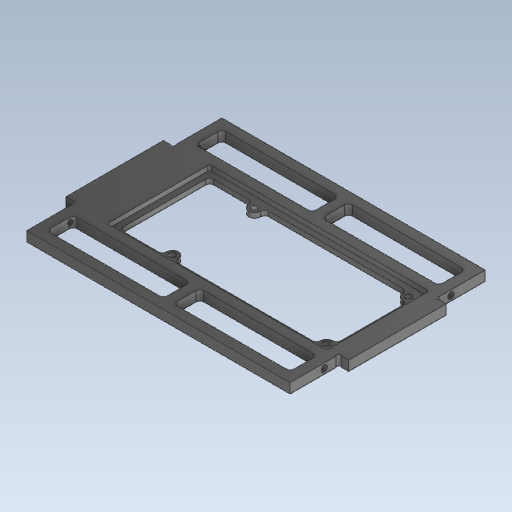
# Autodesk Inventor part: Cockpit_carrier_board_frame
Saved by Autodesk Inventor 2020.4 (Build 244396000, 396)
## iProperties
Created: 2022-01-28
Part Number: Cockpit_carrier_board_frame
Material: アセタール樹脂、黒
Document SubType Name: Modeling
Designer: Masato Kubotera
Density: 1.425 g/cm^3
Appearance: 滑らか - 黒
Author: Masato Kubotera
Autodesk Inventor part; units mm, degrees
ref_plane "YZ Plane" through (0, 0, 0) normal (1, 0, 0) x (0, 1, 0)
derived "Cockpit_side_frame.ipt"
sketch "スケッチ2" plane through (0, 0, 0) normal (0, 1, 0) x (-1, 0, 0)
  line L0 (-28.5, -22.5) -> (86.5, -22.5) construction
  line L1 (86.5, -22.5) -> (86.5, -138.5)
  line L2 (86.5, -96) -> (-28.5, -96) construction
  line L3 (-28.5, -96) -> (-28.5, -22.5) construction
  line L4 (-28.5, -22.5) -> (86.5, -96) construction
  line L5 (86.5, -22.5) -> (-28.5, -96) construction
  line L6 (36.5, -101) -> (36.5, -133.5)
  line L7 (41.5, -138.5) -> (86.5, -138.5)
  arc A0 (62.6349, -70.4) -> (61.15, -71.8849) centre (61.8925, -71.1425) ccw
  arc A1 (71.15, -72.5349) -> (69.6651, -71.05) centre (70.4075, -71.7925) ccw
  line L8 (63.3349, -71.05) -> (69.6651, -71.05)
  line L9 (62.6349, -70.4) -> (70.3651, -70.4)
  line L10 (61.9, -71.1) -> (71.1, -71.1) construction
  arc A2 (63.3349, -71.05) -> (61.85, -72.5349) centre (62.5925, -71.7925) ccw
  line L11 (61.2, -70.45) -> (71.8, -70.45) construction
  line L12 (71.15, -72.5349) -> (71.15, -83.4651)
  line L13 (71.8, -78) -> (61.2, -78) construction
  line L14 (71.85, -71.8849) -> (71.85, -84.1151)
  line L15 (71.1, -71.1) -> (71.1, -84.9) construction
  line L16 (61.85, -72.5349) -> (61.85, -83.4651)
  line L17 (71.8, -70.45) -> (71.8, -85.55) construction
  line L18 (61.15, -71.8849) -> (61.15, -84.1151)
  line L19 (66.5, -70.45) -> (66.5, -85.55) construction
  line L20 (61.9, -84.9) -> (61.9, -71.1) construction
  line L21 (71.1, -71.1) -> (61.9, -84.9) construction
  line L22 (71.8, -70.45) -> (61.2, -85.55) construction
  line L23 (61.2, -70.45) -> (71.8, -85.55) construction
  line L24 (61.2, -85.55) -> (61.2, -70.45) construction
  line L25 (61.9, -71.1) -> (71.1, -84.9) construction
  arc A3 (71.85, -71.8849) -> (70.3651, -70.4) centre (71.1075, -71.1425) ccw
  line L26 (71.1, -84.9) -> (61.9, -84.9) construction
  line L27 (71.8, -85.55) -> (61.2, -85.55) construction
  arc A4 (61.85, -83.4651) -> (63.3349, -84.95) centre (62.5925, -84.2075) ccw
  arc A5 (61.15, -84.1151) -> (62.6349, -85.6) centre (61.8925, -84.8575) ccw
  line L28 (63.3349, -84.95) -> (69.6651, -84.95)
  line L29 (62.6349, -85.6) -> (70.3651, -85.6)
  arc A6 (69.6651, -84.95) -> (71.15, -83.4651) centre (70.4075, -84.2075) ccw
  arc A7 (70.3651, -85.6) -> (71.85, -84.1151) centre (71.1075, -84.8575) ccw
  line L30 (-23.5, -22.5) -> (-28.5, -27.5)
  line L31 (-28.5, -59.25) -> (86.5, -59.25) construction
  line L32 (29, -22.5) -> (29, -96) construction
  line L33 (-23.5, -96) -> (-28.5, -91)
  line L34 (-28.5, -27.5) -> (-28.5, -91)
  line L35 (-21, -25) -> (-26, -25) construction
  line L36 (-26, -25) -> (-26, -93.5) construction
  line L37 (-26, -93.5) -> (-21, -93.5) construction
  line L38 (-21, -93.5) -> (-21, -25) construction
  line L39 (-21, -25) -> (-26, -93.5) construction
  line L40 (-26, -25) -> (-21, -93.5) construction
  line L41 (-26.05, -46.7) -> (-20.95, -46.7)
  line L42 (-20.95, -46.7) -> (-20.95, -71.8)
  line L43 (-20.95, -71.8) -> (-26.05, -71.8)
  line L44 (-26.05, -71.8) -> (-26.05, -46.7)
  line L45 (-26.05, -46.7) -> (-20.95, -71.8) construction
  line L46 (-20.95, -46.7) -> (-26.05, -71.8) construction
  line L47 (-26, -46.75) -> (-21, -46.75) construction
  line L48 (-26, -71.75) -> (-21, -71.75) construction
  line L49 (-23.5, -25) -> (-23.5, -93.5) construction
  circle A8 centre (-23.5, -35) radius 3
  circle A9 centre (-23.5, -35) radius 1.6
  arc A10 (-24.5651, -46.7) -> (-26.05, -48.1849) centre (-25.3075, -47.4425) ccw
  arc A11 (-20.95, -48.1849) -> (-22.4349, -46.7) centre (-21.6925, -47.4425) ccw
  arc A12 (-22.4349, -71.8) -> (-20.95, -70.3151) centre (-21.6925, -71.0575) ccw
  arc A13 (-26.05, -70.3151) -> (-24.5651, -71.8) centre (-25.3075, -71.0575) ccw
  circle A14 centre (-23.5, -83.5) radius 1.6
  circle A15 centre (-23.5, -83.5) radius 3
  line L50 (31.5, -96) -> (36.5, -101)
  line L51 (-23.5, -96) -> (31.5, -96)
  line L52 (79, -67.5) -> (-21, -67.5) construction
  line L53 (-21, -67.5) -> (-21, -62.5) construction
  line L54 (-21, -62.5) -> (79, -62.5) construction
  line L55 (79, -62.5) -> (79, -67.5) construction
  line L56 (79, -67.5) -> (-21, -62.5) construction
  line L57 (-21, -67.5) -> (79, -62.5) construction
  line L58 (-21, -65) -> (79, -65) construction
  line L59 (29, -62.5) -> (29, -67.5) construction
  line L60 (4, -62.5) -> (4, -67.5) construction
  line L61 (54.05, -62.45) -> (3.95, -62.45)
  line L62 (3.95, -62.45) -> (3.95, -67.55)
  line L63 (3.95, -67.55) -> (54.05, -67.55)
  line L64 (54.05, -67.55) -> (54.05, -62.45)
  line L65 (54.05, -62.45) -> (3.95, -67.55) construction
  line L66 (3.95, -62.45) -> (54.05, -67.55) construction
  arc A16 (5.4349, -62.45) -> (3.95, -63.9349) centre (4.6925, -63.1925) ccw
  circle A17 centre (-3.5, -65) radius 3
  circle A18 centre (-3.5, -65) radius 1.6
  line L67 (54, -62.5) -> (54, -67.5) construction
  arc A19 (54.05, -63.9349) -> (52.5651, -62.45) centre (53.3075, -63.1925) ccw
  circle A20 centre (61.5, -65) radius 3
  circle A21 centre (61.5, -65) radius 1.6
  arc A22 (3.95, -66.0651) -> (5.4349, -67.55) centre (4.6925, -66.8075) ccw
  arc A23 (52.5651, -67.55) -> (54.05, -66.0651) centre (53.3075, -66.8075) ccw
  line L68 (-21, -88.5) -> (79, -88.5) construction
  line L69 (79, -88.5) -> (79, -93.5) construction
  line L70 (79, -93.5) -> (-21, -93.5) construction
  line L71 (-21, -93.5) -> (-21, -88.5) construction
  line L72 (-21, -88.5) -> (79, -93.5) construction
  line L73 (79, -88.5) -> (-21, -93.5) construction
  line L74 (-21, -91) -> (79, -91) construction
  line L75 (29, -88.5) -> (29, -93.5) construction
  line L76 (54.05, -91.05) -> (3.95, -91.05)
  line L77 (3.95, -91.05) -> (3.95, -88.45)
  line L78 (3.95, -88.45) -> (54.05, -88.45)
  line L79 (54.05, -88.45) -> (54.05, -91.05)
  line L80 (54.05, -91.05) -> (3.95, -88.45) construction
  line L81 (3.95, -91.05) -> (54.05, -88.45) construction
  line L82 (4, -88.5) -> (4, -91) construction
  line L83 (54, -88.5) -> (54, -91) construction
  line L84 (4, -89.75) -> (54, -89.75) construction
  arc A24 (6.05, -88.45) -> (3.95, -88.45) centre (5, -88.45) ccw
  arc A25 (54.05, -88.45) -> (51.95, -88.45) centre (53, -88.45) ccw
  arc A26 (51.95, -91.05) -> (54.05, -91.05) centre (53, -91.05) ccw
  arc A27 (3.95, -91.05) -> (6.05, -91.05) centre (5, -91.05) ccw
  circle A28 centre (-3.5, -91) radius 3
  circle A29 centre (-3.5, -91) radius 1.6
  circle A30 centre (61.5, -91) radius 3 construction
  circle A31 centre (61.5, -91) radius 1.6 construction
  line L85 (-23.5, -22.5) -> (64.25, -22.5)
  line L86 (64.25, -22.5) -> (64.25, -17.5)
  line L87 (64.25, -17.5) -> (72.25, -17.5)
  line L88 (72.25, -17.5) -> (72.25, -22.5)
  line L89 (72.25, -22.5) -> (79, -22.5)
  line L90 (79, -22.5) -> (79, -17.5)
  line L91 (86.5, -22.5) -> (86.5, -20)
  line L92 (79, -17.5) -> (84, -17.5)
  line L93 (84, -17.5) -> (86.5, -20)
  line L94 (68.25, -17.5) -> (68.25, -22.5) construction
  arc A32 (62.7651, -22.5) -> (64.25, -21.0151) centre (63.5075, -21.7575) ccw
  arc A33 (72.25, -21.0151) -> (73.7349, -22.5) centre (72.9925, -21.7575) ccw
  arc A34 (77.5151, -22.5) -> (79, -21.0151) centre (78.2575, -21.7575) ccw
  line L95 (-16, -88.5) -> (-16, -68.5) construction
  line L96 (-16, -68.5) -> (64, -68.5) construction
  line L97 (64, -68.5) -> (64, -88.5) construction
  line L98 (45.5, -86) -> (-16.5, -86)
  line L99 (-18.5, -84) -> (-18.5, -72)
  line L100 (-16.5, -70) -> (45.5, -70)
  line L101 (47.5, -72) -> (47.5, -84)
  line L102 (47.5, -86) -> (-18.5, -70) construction
  line L103 (-18.5, -86) -> (47.5, -70) construction
  arc A35 (-16.5, -70) -> (-18.5, -72) centre (-16.5, -72) ccw
  arc A36 (-18.5, -84) -> (-16.5, -86) centre (-16.5, -84) ccw
  arc A37 (45.5, -86) -> (47.5, -84) centre (45.5, -84) ccw
  arc A38 (47.5, -72) -> (45.5, -70) centre (45.5, -72) ccw
  line L104 (36.5, -133.5) -> (41.5, -138.5)
  line L105 (44, -131) -> (39, -131) construction
  line L106 (39, -131) -> (39, -96) construction
  line L107 (39, -96) -> (44, -96) construction
  line L108 (44, -96) -> (44, -131) construction
  line L109 (44, -131) -> (39, -96) construction
  line L110 (39, -131) -> (44, -96) construction
  line L111 (41.5, -96) -> (41.5, -131) construction
  line L112 (39, -113.5) -> (44, -113.5) construction
  line L113 (41.5, -107.5) -> (44, -107.5) construction
  line L114 (41.45, -107.45) -> (44.05, -107.45)
  line L115 (44.05, -107.45) -> (44.05, -119.55)
  line L116 (44.05, -119.55) -> (41.45, -119.55)
  line L117 (41.45, -119.55) -> (41.45, -107.45)
  line L118 (41.45, -107.45) -> (44.05, -119.55) construction
  line L119 (44.05, -107.45) -> (41.45, -119.55) construction
  arc A39 (44.05, -109.55) -> (44.05, -107.45) centre (44.05, -108.5) ccw
  arc A40 (42.9349, -107.45) -> (41.45, -108.9349) centre (42.1925, -108.1925) ccw
  arc A41 (44.05, -119.55) -> (44.05, -117.45) centre (44.05, -118.5) ccw
  line L120 (41.5, -119.5) -> (44, -119.5) construction
  arc A42 (41.45, -118.0651) -> (42.9349, -119.55) centre (42.1925, -118.8075) ccw
  line L121 (42.75, -107.5) -> (42.75, -119.5) construction
  circle A43 centre (41.5, -125.5) radius 3 construction
  circle A44 centre (41.5, -125.5) radius 1.6 construction
  circle A45 centre (41.5, -101.5) radius 3
  circle A46 centre (41.5, -101.5) radius 1.6
  circle A47 centre (-13.5, -55) radius 2
  line L122 (39, -131) -> (77.8645, -131) construction
  line L123 (77.8645, -131) -> (77.8645, -136) construction
  line L124 (77.8645, -136) -> (39, -136) construction
  line L125 (39, -136) -> (39, -131) construction
  line L126 (39, -131) -> (77.8645, -136) construction
  line L127 (77.8645, -131) -> (39, -136) construction
  line L128 (39, -133.5) -> (77.8645, -133.5) construction
  line L129 (58.4322, -131) -> (58.4322, -136) construction
  line L130 (58.4322, -133.5) -> (58.4322, -131) construction
  line L131 (50.8822, -130.95) -> (65.9822, -130.95)
  line L132 (65.9822, -130.95) -> (65.9822, -133.55)
  line L133 (65.9822, -133.55) -> (50.8822, -133.55)
  line L134 (50.8822, -133.55) -> (50.8822, -130.95)
  line L135 (50.8822, -130.95) -> (65.9822, -133.55) construction
  line L136 (65.9822, -130.95) -> (50.8822, -133.55) construction
  line L137 (50.9322, -131) -> (50.9322, -133.5) construction
  arc A48 (52.9822, -130.95) -> (50.8822, -130.95) centre (51.9322, -130.95) ccw
  arc A49 (50.8822, -132.0651) -> (52.3672, -133.55) centre (51.6247, -132.8075) ccw
  arc A50 (65.9822, -130.95) -> (63.8822, -130.95) centre (64.9322, -130.95) ccw
  arc A51 (64.4973, -133.55) -> (65.9822, -132.0651) centre (65.2398, -132.8075) ccw
  line L138 (65.9322, -131) -> (65.9322, -133.5) construction
  line L139 (50.9322, -132.25) -> (65.9322, -132.25) construction
  circle A52 centre (72.4322, -133.5) radius 1.6 construction
  circle A53 centre (72.4322, -133.5) radius 3 construction
  circle A54 centre (44.4322, -133.5) radius 3
  circle A55 centre (44.4322, -133.5) radius 1.6
  line L140 (48.5, -96) -> (77, -96)
  line L141 (79, -98) -> (79, -126.5)
  line L142 (77, -128.5) -> (48.5, -128.5)
  line L143 (46.5, -126.5) -> (46.5, -98)
  line L144 (46.5, -96) -> (79, -128.5) construction
  line L145 (79, -96) -> (46.5, -128.5) construction
  arc A56 (48.5, -96) -> (46.5, -98) centre (48.5, -98) ccw
  arc A57 (46.5, -126.5) -> (48.5, -128.5) centre (48.5, -126.5) ccw
  arc A58 (77, -128.5) -> (79, -126.5) centre (77, -126.5) ccw
  arc A59 (79, -98) -> (77, -96) centre (77, -98) ccw
  line L146 (79, -91.1738) -> (84, -91.1738) construction
  line L147 (84, -91.1738) -> (84, -136) construction
  line L148 (84, -136) -> (79, -136) construction
  line L149 (79, -136) -> (79, -91.1738) construction
  line L150 (79, -91.1738) -> (84, -136) construction
  line L151 (84, -91.1738) -> (79, -136) construction
  line L152 (81.5, -91.1738) -> (81.5, -136) construction
  circle A60 centre (81.5, -93.6738) radius 1.475
  circle A61 centre (81.5, -98.6738) radius 1.475
  circle A62 centre (81.5, -103.6738) radius 1.475
  circle A63 centre (81.5, -133.5) radius 1.6
  arc A64 (84, -91.1738) -> (79, -91.1738) centre (81.5, -133.5) ccw construction
  arc A65 (84.0111, -91.0742) -> (78.9889, -91.0742) centre (81.5, -133.5) ccw construction
  line L153 (86.5, -133.5) -> (81.5, -138.5)
  arc A66 (79, -131) -> (84, -136) centre (81.5, -133.5) ccw construction
  line L154 (79, -65) -> (84, -65) construction
  line L155 (84, -65) -> (84, -91) construction
  line L156 (84, -91) -> (79, -91) construction
  line L157 (79, -91) -> (79, -65) construction
  line L158 (79, -65) -> (84, -91) construction
  line L159 (84, -65) -> (79, -91) construction
  line L160 (79, -78) -> (84, -78) construction
  line L161 (81.5, -65) -> (81.5, -91) construction
  line L162 (79, -73) -> (84, -73) construction
  line L163 (78.95, -72.95) -> (86.5, -72.95)
  line L164 (84.05, -72.95) -> (84.05, -83.05) construction
  line L165 (84.05, -83.05) -> (78.95, -83.05)
  line L166 (78.95, -83.05) -> (78.95, -72.95)
  line L167 (78.95, -72.95) -> (84.05, -83.05) construction
  line L168 (84.05, -72.95) -> (78.95, -83.05) construction
  arc A67 (80.4349, -72.95) -> (78.95, -74.4349) centre (79.6925, -73.6925) ccw
  arc A68 (78.95, -81.5651) -> (80.4349, -83.05) centre (79.6925, -82.3075) ccw
  line L169 (79, -83) -> (84, -83) construction
  circle A69 centre (81.5, -68) radius 1.6
  circle A70 centre (81.5, -68) radius 3
  circle A71 centre (81.5, -88) radius 1.6
  circle A72 centre (81.5, -88) radius 3
  line L170 (84.05, -83.05) -> (86.5, -83.05)
  circle A73 centre (81.5, -133.5) radius 3
  line L171 (75.625, -22.5) -> (75.625, -27.147) construction
  line L172 (60.875, -22.5) -> (60.875, -27.147) construction
  line L173 (64.25, -22.5) -> (72.25, -22.5)
  point P0 (0, 0)
  point P1 (29, -59.25)
  point P2 (-25.7227, -96)
  point P3 (61.85, -71.05)
  point P4 (61.15, -70.4)
  point P5 (66.5, -78)
  point P6 (-23.5, -59.25)
  point P7 (29, -65)
  point P8 (29, -91)
  point P9 (29, -89.75)
  point P10 (29, -89.75)
  point P11 (52.5, -22)
  point P12 (14.5, -78)
  point P13 (-18.5, -61)
  point P14 (47.5, -61)
  point P15 (41.5, -113.5)
  point P16 (42.75, -113.5)
  point P17 (58.4322, -133.5)
  point P18 (58.4322, -132.25)
  point P19 (62.75, -112.25)
  point P20 (81.5, -113.5869)
  point P21 (81.5, -78)
  dimension "d1" = 67.5
  dimension "d2" = 5
  measures "d1" vertical distance of L52.start point (0, 0)
  measures "d2" distance of L54.end L52.start
ref_plane "作業平面1" through (0, 0, -67.5) normal (0, 0, 1) x (1, 0, 0)
sketch "スケッチ3" plane through (0, 0, -67.5) normal (0, 0, 1) x (1, 0, 0)
  line L0 (21, 0) -> (-79, 0) construction
  line L1 (-79, 0) -> (-79, -135)
  line L2 (-79, -135) -> (21, -135) construction
  line L3 (21, -135) -> (21, 0)
  line L4 (21, 0) -> (-79, -135) construction
  line L5 (-79, 0) -> (21, -135) construction
  line L6 (-4, 0) -> (-4, 5)
  line L7 (-4, 5) -> (-54, 5)
  line L8 (-54, 5) -> (-54, 0)
  arc A0 (-4, 1.4849) -> (-2.5151, 0) centre (-3.2575, 0.7425) ccw
  line L9 (-29, 0) -> (-29, -135) construction
  line L10 (21, -67.5) -> (-79, -67.5) construction
  arc A1 (-55.4849, 0) -> (-54, 1.4849) centre (-54.7425, 0.7425) ccw
  line L11 (-2.75, -117.5) -> (-55.25, -117.5)
  line L12 (-55.25, -117.5) -> (-55.25, -5)
  line L13 (-55.25, -5) -> (-2.75, -5)
  line L14 (-2.75, -5) -> (-2.75, -117.5)
  line L15 (-2.75, -117.5) -> (-55.25, -5) construction
  line L16 (-55.25, -117.5) -> (-2.75, -5) construction
  line L17 (-29, -5) -> (-29, -117.5) construction
  line L18 (-4, -6.25) -> (-54, -6.25) construction
  line L19 (-54, -6.25) -> (-54, -116.25) construction
  line L20 (-54, -116.25) -> (-4, -116.25) construction
  line L21 (-4, -116.25) -> (-4, -6.25) construction
  line L22 (-4, -6.25) -> (-54, -116.25) construction
  line L23 (-54, -6.25) -> (-4, -116.25) construction
  line L24 (-8, -89.25) -> (-50, -89.25) construction
  line L25 (-50, -89.25) -> (-50, -10.25) construction
  line L26 (-50, -10.25) -> (-8, -10.25) construction
  line L27 (-8, -10.25) -> (-8, -89.25) construction
  line L28 (-8, -89.25) -> (-50, -10.25) construction
  line L29 (-50, -89.25) -> (-8, -10.25) construction
  circle A2 centre (-50, -10.25) radius 1.6
  circle A3 centre (-50, -89.25) radius 1.6
  circle A4 centre (-8, -10.25) radius 1.6
  circle A5 centre (-8, -89.25) radius 1.6
  arc A6 (-50.15, -13.2462) -> (-47.0038, -10.1) centre (-50, -10.25) ccw
  line L30 (-45.0063, -8) -> (-12.9937, -8)
  arc A7 (-50.15, -92.2462) -> (-50.15, -86.2538) centre (-50, -89.25) ccw
  line L31 (-52.25, -94.2437) -> (-52.25, -112.5)
  line L32 (-50.25, -114.5) -> (-7.75, -114.5)
  line L33 (-52.25, -15.2437) -> (-52.25, -84.2563)
  arc A8 (-10.9962, -10.1) -> (-7.85, -13.2462) centre (-8, -10.25) ccw
  arc A9 (-7.85, -86.2538) -> (-7.85, -92.2462) centre (-8, -89.25) ccw
  line L34 (-5.75, -94.2437) -> (-5.75, -112.5)
  line L35 (-5.75, -15.2437) -> (-5.75, -84.2563)
  arc A10 (-45.0063, -8) -> (-47.0038, -10.1) centre (-45.0063, -10) ccw
  arc A11 (-50.15, -13.2462) -> (-52.25, -15.2437) centre (-50.25, -15.2437) ccw
  arc A12 (-52.25, -84.2563) -> (-50.15, -86.2538) centre (-50.25, -84.2563) ccw
  arc A13 (-50.15, -92.2462) -> (-52.25, -94.2437) centre (-50.25, -94.2437) ccw
  arc A14 (-52.25, -112.5) -> (-50.25, -114.5) centre (-50.25, -112.5) ccw
  arc A15 (-7.75, -114.5) -> (-5.75, -112.5) centre (-7.75, -112.5) ccw
  arc A16 (-5.75, -94.2437) -> (-7.85, -92.2462) centre (-7.75, -94.2437) ccw
  arc A17 (-7.85, -86.2538) -> (-5.75, -84.2563) centre (-7.75, -84.2563) ccw
  arc A18 (-10.9962, -10.1) -> (-12.9937, -8) centre (-12.9937, -10) ccw
  arc A19 (-5.75, -15.2437) -> (-7.85, -13.2462) centre (-7.75, -15.2437) ccw
  line L36 (-79, 0) -> (-55.4849, 0)
  line L37 (-2.5151, 0) -> (21, 0)
  line L38 (-4, -135) -> (-4, -140)
  line L39 (-4, -140) -> (-54, -140)
  line L40 (-54, -140) -> (-54, -135)
  arc A20 (-2.5151, -135) -> (-4, -136.4849) centre (-3.2575, -135.7425) ccw
  line L41 (-79, -135) -> (-55.4849, -135)
  line L42 (-2.5151, -135) -> (21, -135)
  line L43 (14, -65) -> (4.25, -65)
  line L44 (2.25, -63) -> (2.25, -7)
  line L45 (4.25, -5) -> (14, -5)
  line L46 (16, -7) -> (16, -63)
  line L47 (16, -65) -> (2.25, -5) construction
  line L48 (2.25, -65) -> (16, -5) construction
  arc A21 (4.25, -5) -> (2.25, -7) centre (4.25, -7) ccw
  arc A22 (2.25, -63) -> (4.25, -65) centre (4.25, -63) ccw
  arc A23 (14, -65) -> (16, -63) centre (14, -63) ccw
  arc A24 (16, -7) -> (14, -5) centre (14, -7) ccw
  line L49 (14, -70) -> (4.25, -70)
  line L50 (2.25, -72) -> (2.25, -128)
  line L51 (4.25, -130) -> (14, -130)
  line L52 (16, -128) -> (16, -72)
  arc A25 (2.25, -128) -> (4.25, -130) centre (4.25, -128) ccw
  arc A26 (4.25, -70) -> (2.25, -72) centre (4.25, -72) ccw
  arc A27 (16, -72) -> (14, -70) centre (14, -72) ccw
  arc A28 (14, -130) -> (16, -128) centre (14, -128) ccw
  line L53 (-72, -65) -> (-62.25, -65)
  line L54 (-60.25, -63) -> (-60.25, -7)
  line L55 (-62.25, -5) -> (-72, -5)
  line L56 (-74, -7) -> (-74, -63)
  arc A29 (-60.25, -7) -> (-62.25, -5) centre (-62.25, -7) ccw
  arc A30 (-62.25, -65) -> (-60.25, -63) centre (-62.25, -63) ccw
  arc A31 (-72, -5) -> (-74, -7) centre (-72, -7) ccw
  line L57 (-62.25, -130) -> (-72, -130)
  arc A32 (-62.25, -130) -> (-60.25, -128) centre (-62.25, -128) ccw
  arc A33 (-74, -128) -> (-72, -130) centre (-72, -128) ccw
  line L58 (-74, -128) -> (-74, -72)
  line L59 (-60.25, -72) -> (-60.25, -128)
  arc A34 (-72, -70) -> (-74, -72) centre (-72, -72) ccw
  line L60 (-72, -70) -> (-62.25, -70)
  arc A35 (-60.25, -72) -> (-62.25, -70) centre (-62.25, -72) ccw
  arc A36 (-54, -136.4849) -> (-55.4849, -135) centre (-54.7425, -135.7425) ccw
  arc A37 (-74, -63) -> (-72, -65) centre (-72, -63) ccw
  point P0 (0, 0)
  point P1 (-54, 1.4849)
  point P2 (-55.4849, 0)
  point P3 (-29, -61.25)
  point P4 (-29, -61.25)
  point P5 (-29, -49.75)
  point P6 (-52.25, -12.2343)
  point P7 (-48.0157, -8)
  point P8 (-52.25, -91.2343)
  point P9 (-52.25, -87.2657)
  point P10 (-52.25, -114.5)
  point P11 (-5.75, -12.2343)
  point P12 (-9.9843, -8)
  point P13 (-5.75, -91.2343)
  point P14 (-5.75, -87.2657)
  point P15 (-5.75, -114.5)
  point P16 (9.125, -35)
  dimension "d4" = 5
  dimension "d5" = 135
  dimension "d6" = 1.05
  dimension "d27" = 110
  dimension "d28" = 50
  dimension "d29" = 42
  dimension "d30" = 4
  dimension "d31" = 79
  dimension "d32" = 1.25
  dimension "d33" = 1.25
  dimension "d34" = 1.25
  dimension "d35" = 3.2
  dimension "d36" = 3.2
  dimension "d38" = 3
  dimension "d39" = 3
  dimension "d40" = 3
  dimension "d41" = 3
  dimension "d42" = 3
  dimension "d43" = 2
  dimension "d44" = 5
  dimension "d45" = 0
  dimension "d46" = 5
  dimension "d47" = 5
  dimension "d48" = 5
  dimension "d49" = 2.5
  dimension "d50" = 2
  constraints: 122 end point, 77 point on circle, 68 symmetric about line, 38 centre point, 28 tangent, 26 point on line, 15 midpoint, 12 equal radius, 12 parallel, 10 coincident, 8 perpendicular, 6 horizontal, 3 collinear, 1 vertical, 19 other
  measures "d4" distance of L6.start L6.end
  measures "d5" distance of L2.end L0.start
  measures "d6" radius of A0
  measures "d27" distance of L20.end L18.start
  measures "d28" distance of L18.start L18.end
  measures "d29" distance of L25.end L26.end
  measures "d30" horizontal distance of L18.end L25.end
  measures "d31" distance of L24.end L25.end
  measures "d32" horizontal distance of L12.end L18.end
  measures "d33" horizontal distance of L11.end L19.end
  measures "d34" horizontal distance of L12.end L18.end
  measures "d35" diameter of A2
  measures "d36" diameter of A3
  measures "d38" horizontal distance of L11.end point (-52.25, -114.5)
  measures "d39" horizontal distance of L11.end point (-52.25, -114.5)
  measures "d40" vertical distance of point (-48.016, -8) L12.end
  measures "d41" radius of A7
  measures "d42" radius of A6
  measures "d43" radius of A10
  measures "d44" vertical distance of L0.start L13.end
  measures "d45" horizontal distance of L9.start L17.start
  measures "d46" horizontal distance of L0.start L48.end
  measures "d47" distance of L13.end L47.end
  measures "d48" horizontal distance of L48.end L0.start
  measures "d49" vertical distance of L10.start L47.start
  measures "d50" radius of A21
extrude "押し出し1" add sketch "スケッチ3" along normal blind 5 contours L36 A1 L8 L7 L6 A0 L37 L3 L42 A20 L38 L39 L40 A36 L41 L1
hole "穴1" at (-61.5, 0, -65) at (3.5, 0, -65) direction (0, -1, 0) diameter 3.242 depth 5 tip angle 118 thread size "M4x0.7" class "6H" standard "ISO Metric profile"
extrude "押し出し2" add sketch "スケッチ3" along normal blind 2.5 contours L11 L12 L13 L14
fillet "フィレット1" radius 1 4 edges at (-55.25, -117.5, -63.75) (-2.75, -117.5, -63.75) (-2.75, -5, -63.75) (-55.25, -5, -63.75)
ref_plane "作業平面2" through (0, -67.5, 0) normal (0, 1, 0) x (-1, 0, 0)
mirror "ミラー1" about plane through (0, -67.5, 0) normal (0, 1, 0) of "穴1"
equation "\"d33\" = d32"
equation "\"d34\" = d32"
equation "\"d38\" = d39"
equation "\"d40\" = d39"
equation "\"d47\" = d46"
equation "\"d49\" = 0.5 * d48"
equation "\"d7\" = d2"
equation "\"d3\" = -d1"
